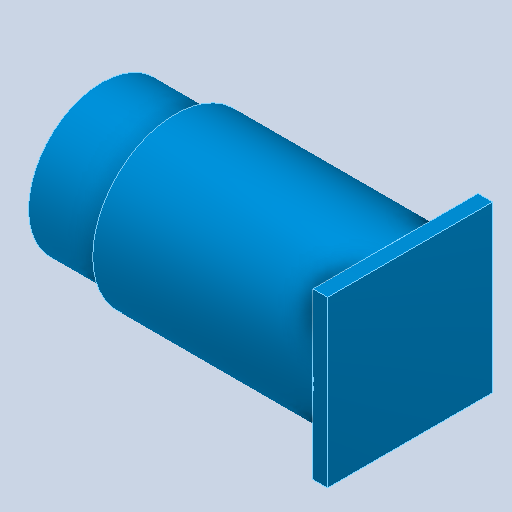
# Autodesk Inventor part: temporary_motor
Saved by Autodesk Inventor 2025.3 (Build 293356030, 356C)
## iProperties
Created: 2025-08-09
Part Number: temporary_motor
Material: 알루미늄 6061
Document SubType Name: Modeling
Designer: LeeJinWon
Density: 2.7 g/cm^3
Appearance: 알루미늄 - 평지
Project: Robot Arm
Mass: 2779.03 g
Surface Area: 630.623 cm^2
Volume: 1029.27 cm^3
Author: LeeJinWon
Autodesk Inventor part; units mm, degrees
ref_plane "YZ Plane" through (0, 0, 0) normal (1, 0, 0) x (0, 1, 0)
ref_plane "XZ Plane" through (0, 0, 0) normal (0, 1, 0) x (-1, 0, 0)
ref_plane "XY Plane" through (0, 0, 0) normal (0, 0, 1) x (1, 0, 0)
sketch "스케치1" plane through (0, 0, 0) normal (1, 0, 0) x (0, 1, 0)
  circle A0 centre (0, 0) radius 45
  dimension "d0" = 90
  constraints: 1 centre point, 1 coincident
  measures "d0" diameter of A0
extrude "돌출1" add sketch "스케치1" along normal mid plane 160
sketch "스케치2" plane through (80, 0, 0) normal (1, 0, 0) x (0, 0, -1)
  line L0 (-45, 45) -> (45, 45)
  line L1 (45, 45) -> (45, -45)
  line L2 (45, -45) -> (-45, -45)
  line L3 (-45, -45) -> (-45, 45)
  line L4 (-45, 45) -> (45, -45) construction
  line L5 (45, 45) -> (-45, -45) construction
  circle A0 centre (0, 0) radius 45 projected
  point P0 (0, 0)
  constraints: 12 end point, 3 tangent, 2 midpoint, 2 parallel, 2 perpendicular, 1 horizontal
extrude "돌출2" add sketch "스케치2" along normal blind 8
sketch "스케치4" plane through (-80, 0, 0) normal (-1, 0, 0) x (0, 0, 1)
  circle A0 centre (0, 0) radius 40
  circle A1 centre (0, 0) radius 45 projected
  dimension "d15" = 80
  constraints: 1 centre point, 1 coincident
  measures "d15" diameter of A0
extrude "돌출3" cut sketch "스케치4" against normal blind 40
sketch "스케치3" plane through (88, 0, 0) normal (1, 0, 0) x (0, 0, -1)
  line L0 (-36.5, 36.5) -> (36.5, 36.5) construction
  line L1 (36.5, 36.5) -> (36.5, -36.5) construction
  line L2 (36.5, -36.5) -> (-36.5, -36.5) construction
  line L3 (-36.5, -36.5) -> (-36.5, 36.5) construction
  line L4 (-36.5, 36.5) -> (36.5, -36.5) construction
  line L5 (36.5, 36.5) -> (-36.5, -36.5) construction
  point P0 (0, 0)
  dimension "d6" = 73
  dimension "d7" = 73
  constraints: 12 end point, 2 midpoint, 2 parallel, 1 horizontal, 1 perpendicular
  measures "d6" distance of L1.end L2.end
  measures "d7" distance of L0.end L1.end
